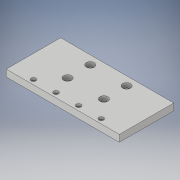
# Autodesk Inventor part: base_part
Saved by Autodesk Inventor 2019 (Build 230136000, 136)
## iProperties
Created: 2019-03-08
Part Number: base_part
Material: Generic
Document SubType Name: Modeling
Designer: Wilson Lab
Density: 1 g/cm^3
Appearance: Default
Author: Wilson Lab
Autodesk Inventor part; units mm, degrees
ref_plane "YZ Plane" through (0, 0, 0) normal (1, 0, 0) x (0, 1, 0)
ref_plane "XZ Plane" through (0, 0, 0) normal (0, 1, 0) x (-1, 0, 0)
ref_plane "XY Plane" through (0, 0, 0) normal (0, 0, 1) x (1, 0, 0)
sketch "Sketch1" plane through (0, 0, 0) normal (0, 1, 0) x (-1, 0, 0)
  line L0 (38, 79) -> (-38, 79)
  line L1 (-38, 79) -> (-38, -79)
  line L2 (-38, -79) -> (38, -79)
  line L3 (38, -79) -> (38, 79)
  line L4 (0, 0) -> (38, 0) construction
  line L5 (0, 0) -> (0, -79) construction
  dimension "d0" = 158
  dimension "d1" = 76
  constraints: 12 end point, 3 perpendicular, 2 midpoint, 2 parallel, 1 horizontal
  measures "d0" distance of L2.end L0.start
  measures "d1" distance of L1.end L2.end
extrude "Extrusion1" add sketch "Sketch1" along normal blind 9.525
sketch "Sketch2" plane through (0, 0, 0) normal (0, -1, 0) x (1, 0, 0)
  line L0 (-38, 79) -> (38, 79) construction
  line L1 (-38, -79) -> (-38, 79) construction
  line L2 (38, -79) -> (-38, -79) construction
  line L3 (38, 79) -> (38, -79) construction
  line L4 (-6, -25.4) -> (-6, 25.4) construction
  line L5 (-38, 0) -> (38, 0) construction
  line L6 (25.75, -25.4) -> (25.75, 25.4) construction
  point P0 (0, 0)
  point P1 (-6, 0)
  point P2 (25.75, 0)
  dimension "d4" = 50.8
  dimension "d5" = 50.8
  dimension "d6" = 31.75
  dimension "d16" = 32
  constraints: 6 end point, 4 coincident, 4 midpoint, 2 point on line, 2 vertical
  measures "d4" distance of L4.start L4.end
  measures "d5" distance of L6.start L6.end
  measures "d6" distance between parallel lines of L6 L4
  measures "d16" distance between parallel lines of L1 L4
hole "Hole1" at (-6, 0, 25.4) at (25.75, 0, 25.4) at (25.75, 0, -25.4) at (-6, 0, -25.4) direction (0, 1, 0) diameter 6.756 end through all counterbore diameter 11.113 counterbore depth 6.35 clearance for "Socket Head Cap Screw" size "1/4" standard "Ansi Unified Screw Threads"
sketch "Sketch3" plane through (0, 9.525, 0) normal (0, 1, 0) x (1, 0, 0)
  line L0 (38, -79) -> (38, 79) construction
  line L1 (38, 79) -> (-38, 79) construction
  line L2 (-38, 79) -> (-38, -79) construction
  line L3 (-38, -79) -> (38, -79) construction
  line L4 (-31.65, 79) -> (-31.65, -79) construction
  point P0 (0, 0)
  point P1 (-31.65, 47.4)
  point P2 (-31.65, 15.8)
  point P3 (-31.65, -47.4)
  point P4 (-31.65, -15.8)
  dimension "d17" = 6.35
  dimension "d19" = 31.6
  dimension "d20" = 31.6
  dimension "d21" = 31.6
  dimension "d22" = 31.6
  dimension "d23" = 31.6
  constraints: 6 point on line, 2 end point, 1 perpendicular
  measures "d17" distance between parallel lines of L4 L2
  measures "d19" distance from line of L1 point (-31.65, 47.4)
  measures "d20" distance of point (-31.65, 47.4) point (-31.65, 15.8)
  measures "d21" distance from line of point (-31.65, -47.4) L3
  measures "d22" distance of point (-31.65, -15.8) point (-31.65, -47.4)
  measures "d23" distance of point (-31.65, -15.8) point (-31.65, 15.8)
hole "Hole2" at (-31.65, 9.525, -47.4) at (-31.65, 9.525, -15.8) at (-31.65, 9.525, 47.4) at (-31.65, 9.525, 15.8) direction (0, -1, 0) diameter 6.756 end through all counterbore diameter 11.113 counterbore depth 6.35 clearance for "Socket Head Cap Screw" size "1/4" standard "Ansi Unified Screw Threads"
body "Solid1"
